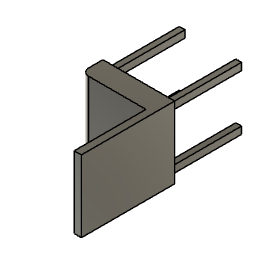
CHAIR v1 (Autodesk Fusion 360 design; units mm, degrees)
Autodesk Fusion 360 part; units mm, degrees
sketch "Sketch1" plane through (0, 0, 0) normal (0, 1, 0) x (1, 0, 0)
  line L0 (0, 0) -> (50, 0)
  line L1 (50, 0) -> (50, -50)
  line L2 (50, -50) -> (0, -50)
  line L3 (0, -50) -> (0, 0)
  dimension "d1" = 50
  dimension "d2" = 50
  constraint horizontal L0
  constraint vertical L1
  constraint horizontal L2
  constraint vertical L3
  constraint coincident L0.start L3.end
  measures "d1" distance of L0.start L0.end
  measures "d2" distance of L0.start L2.end
extrude "Extrude1" add sketch "Sketch1" along normal blind 15
sketch "Sketch2" plane through (0, 15, 0) normal (0, 1, 0) x (-1, 0, 0)
  line L0 (0, 50) -> (-50, 50)
  line L1 (-50, 50) -> (-50, 0)
  line L2 (-50, 0) -> (0, 0)
  line L3 (0, 0) -> (0, 50)
  line L4 (-25, 50) -> (-25, 0) construction
  line L5 (0, 25) -> (-50, 25) construction
  line L6 (-46.6959, 41.7465) -> (-42.6959, 41.7465)
  line L7 (-42.6959, 41.7465) -> (-42.6959, 46.7465)
  line L8 (-42.6959, 46.7465) -> (-46.6959, 46.7465)
  line L9 (-46.6959, 46.7465) -> (-46.6959, 41.7465)
  line L10 (-42.6959, 3.2535) -> (-46.6959, 3.2535)
  line L11 (-46.6959, 3.2535) -> (-46.6959, 8.2535)
  line L12 (-46.6959, 8.2535) -> (-42.6959, 8.2535)
  line L13 (-42.6959, 8.2535) -> (-42.6959, 3.2535)
  line L14 (-3.3041, 41.7465) -> (-7.3041, 41.7465)
  line L15 (-3.3041, 46.7465) -> (-3.3041, 41.7465)
  line L16 (-7.3041, 41.7465) -> (-7.3041, 46.7465)
  line L17 (-7.3041, 46.7465) -> (-3.3041, 46.7465)
  line L18 (-7.3041, 8.2535) -> (-7.3041, 3.2535)
  line L19 (-3.3041, 8.2535) -> (-7.3041, 8.2535)
  line L20 (-3.3041, 3.2535) -> (-3.3041, 8.2535)
  line L21 (-7.3041, 3.2535) -> (-3.3041, 3.2535)
  dimension "d5" = 5
  dimension "d6" = 4
  constraint midpoint L0 L4.start
  constraint midpoint L2 L4.end
  constraint midpoint L3 L5.start
  constraint midpoint L1 L5.end
  constraint horizontal L6
  constraint vertical L7
  constraint horizontal L8
  constraint vertical L9
  constraint symmetric L5 L6.start L11.end
  constraint symmetric L5 L6.end L12.end
  constraint symmetric L5 L7.end L10.start
  constraint symmetric L5 L8.end L10.end
  constraint symmetric L4 L6.start L14.start
  constraint symmetric L4 L6.end L14.end
  constraint symmetric L4 L7.end L16.end
  constraint symmetric L4 L8.end L15.start
  constraint symmetric L4 L10.start L18.end
  constraint symmetric L4 L10.end L20.start
  constraint symmetric L4 L11.end L19.start
  constraint symmetric L4 L12.end L18.start
  measures "d5" distance of L6.start L8.end
  measures "d6" distance of L6.start L6.end
extrude "Extrude2" add sketch "Sketch2" along normal blind 50 contours L6 L7 L8 L9 | L10 L11 L12 L13 | L14 L15 L16 L17 | L18 L19 L20 L21
fillet "Fillet1" radius 5 1 edges at (0, 0, 25)
sketch "Sketch3" plane through (0, 0, 0) normal (0, -1, 0) x (1, 0, 0)
  line L0 (5, 50) -> (5, 0)
  line L1 (5, 0) -> (50, 0)
  line L2 (50, 0) -> (50, 50)
  line L3 (50, 50) -> (5, 50)
  line L4 (50, 0) -> (45, 0)
  line L5 (45, 0) -> (45, 50)
  line L6 (45, 50) -> (50, 50)
  line L7 (50, 50) -> (50, 0)
  dimension "d11" = 5
  dimension "d12" = 50
  constraint horizontal L4
  constraint vertical L5
  constraint horizontal L6
  constraint vertical L7
  constraint coincident L1.end L2.start
  measures "d11" distance of L1.end L4.end
  measures "d12" distance of L1.end L2.end
extrude "Extrude3" add sketch "Sketch3" along normal blind 50 contours L1 L2 L3 L4 L5 L6 L7
